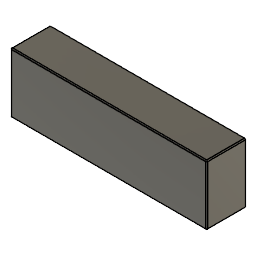
imu_box_v5 (Autodesk Fusion 360 design; units mm, degrees)
Autodesk Fusion 360 part; units mm, degrees
note: some values were not read from the file. Set by a fixed rule: which sketch regions a step uses.
sketch "Sketch1" plane through (0, 0, 0) normal (0, 1, 0) x (1, 0, 0)
  line L0 (0, 0) -> (95, 0)
  line L1 (95, 0) -> (95, -25)
  line L2 (95, -25) -> (0, -25)
  line L3 (0, -25) -> (0, 0)
  line L4 (98, 3) -> (98, -28)
  line L5 (98, -28) -> (-3, -28)
  line L6 (-3, -28) -> (-3, 3)
  line L7 (-3, 3) -> (98, 3)
  dimension "d1" = 95
  dimension "d2" = 25
  dimension "d3" = -3
  constraint horizontal L0
  constraint vertical L1
  constraint horizontal L2
  constraint vertical L3
  constraint coincident L0.start L3.end
  measures "d1" distance of L1.end L2.end
  measures "d2" distance of L0.end L1.end
extrude "Extrude1" add sketch "Sketch1" along normal blind 20 makes body 1
extrude "Extrude2" add sketch "Sketch1" along normal blind 3 contours L0 L1 L2 L3 bodies 1
ref_plane "WorkPlane1" through (47.5, 10, 12.5) normal (0, 0, 1) x (1, 0, 0)
ref_plane "WorkPlane2" through (47.5, 10, 12.5) normal (1, 0, 0) x (0, 0, -1)
sketch "Sketch3" plane through (47.5, 0, 0) normal (1, 0, 0) x (0, 1, 0)
  line L0 (20, 28) -> (0, 28)
  line L1 (0, 28) -> (0, -3)
  line L2 (0, -3) -> (20, -3)
  line L3 (20, -3) -> (20, 0)
  line L4 (20, 0) -> (3, 0)
  line L5 (3, 0) -> (3, 25)
  line L6 (3, 25) -> (20, 25)
  line L7 (20, 25) -> (20, 28)
  circle A0 centre (12.8865, 25) radius 0.75
  circle A1 centre (12.8865, 25) radius 0.9942
  arc A2 (12.1481, 24.8686) -> (20, 21.2966) centre (16.9616, 25.0336) ccw
  arc A3 (13.6365, 25) -> (20, 25) centre (16.8183, 27.2777) ccw
  line L8 (23.2, 12.5) -> (-3.2, 12.5)
  line L9 (20, 28) -> (20, -3)
  line L10 (20, 28) -> (16, 28)
  line L11 (16, 28) -> (16, -3)
  line L12 (20, -3) -> (16, -3)
  arc A4 (20, 0) -> (13.6365, 0) centre (16.8183, -2.2777) ccw
  arc A5 (20, 3.7034) -> (12.1481, 0.1314) centre (16.9616, -0.0336) ccw
  circle A6 centre (12.8865, 0) radius 0.75
  circle A7 centre (12.8865, 0) radius 0.9942
  dimension "d8" = 1.5
  constraint coincident L6 A0.centre
  constraint coincident A0 A2.start
  constraint coincident A0 A3.start
  constraint concentric A0 A1
  constraint coincident L6.end L7.start
  constraint coincident L6 A3.start
  constraint coincident L0.start L7.end
  constraint coincident L2.end L3.start
  constraint coincident A2.end L9
  constraint perpendicular L7 L10
  constraint perpendicular L10 L11
  constraint symmetric A0 L8 A6
  constraint symmetric A1 L8 A7
  constraint symmetric A2.end L8 A5.start
  constraint symmetric A2 L8 A5
  constraint symmetric A3 L8 A4
  constraint symmetric A3.start L8 A4.end
  constraint symmetric A2.start L8 A5.end
  constraint symmetric L8 L6.end L3.end
  measures "d8" diameter of A0
extrude "Extrude9" cut sketch "Sketch3" along normal mid plane 95 contours L6 A1 A3 | L6 A0 A1 | A0 A1 A2 A3 | L6 A0 | L6 A0 | L6 A0 A1 A2 | L4 A5 A6 A7 | L4 A6 A7 | A4 A5 A6 A7 | L4 A4 A7 | L4 A6 | L4 A6 bodies 1
extrude "Extrude10" add sketch "Sketch3" along normal blind 4 from surface at 20 separate body contours A2 A3 L9 L11 | A1 A2 A3 L11 | A0 A1 A2 A3 | L6 A0 | L6 A0 | L9 L11 A4 A5 | L11 A4 A5 A7 | A4 A5 A6 A7 | L4 A6 | L4 A6 makes body 2 at (70.1667, 12.334, 23.6987) makes body 3 at (70.1667, 18.5562, 4.5111)
extrude "Extrude11" add sketch "Sketch3" along normal blind 4 from surface at -20 separate body contours A2 A3 L9 L11 | A1 A2 A3 L11 | A0 A1 A2 A3 | L6 A0 | L6 A0 | L9 L11 A4 A5 | L11 A4 A5 A7 | A4 A5 A6 A7 | L4 A6 | L4 A6 makes body 4 at (30.1667, 18.5562, 4.5111) makes body 5 at (30.1667, 12.334, 23.6987)
extrude "Extrude12" add sketch "Sketch3" along normal mid plane 101 separate body contours L0 L6 L7 L9 L10 L11 | L6 A3 L11 | A2 A3 L9 L11 | A2 L8 L9 L11 | L8 L9 L11 A5 | L9 L11 A4 A5 | L2 L3 L4 L9 L11 L12 | L4 L11 A4 makes body 6
sketch "Sketch8" plane through (0, 16, 0) normal (0, -1, 0) x (1, 0, 0)
  line L0 (-3, -3) -> (98, -3)
  line L1 (98, -3) -> (98, 28)
  line L2 (98, 28) -> (-3, 28)
  line L3 (-3, 28) -> (-3, -3)
  line L4 (0, 10) -> (2.4867, 10)
  line L5 (2.4867, 10) -> (2.4867, 15)
  line L6 (2.4867, 15) -> (0, 15)
  line L7 (0, 15) -> (0, 10)
  line L8 (95, 10) -> (93, 10)
  line L9 (93, 10) -> (93, 15)
  line L10 (93, 15) -> (95, 15)
  line L11 (95, 10) -> (95, 15)
  constraint perpendicular L3 L4
  constraint perpendicular L4 L5
  constraint perpendicular L5 L6
  constraint perpendicular L4 L7
  constraint perpendicular L1 L8
  constraint perpendicular L8 L9
  constraint perpendicular L9 L10
  constraint perpendicular L10 L11
extrude "Extrude13" add sketch "Sketch8" along normal blind 2 contours L4 L5 L6 L7 | L8 L9 L10 L11 bodies 6
fillet "Fillet5" radius 0.5 4 edges at (47.5, 20, 28) (98, 20, 12.5) (47.5, 20, -3) (-3, 20, 12.5) on bodies 6
fillet "Fillet6" radius 1 2 edges at (47.5, 13.8807, 25) (47.5, 13.8807, 0) on bodies 1
fillet "Fillet7" radius 0.5 8 edges at (-3, 10, 28) (-3, 0, 12.5) (-3, 10, -3) (47.5, 0, -3) (47.5, 0, 28) (98, 0, 12.5) (98, 10, -3) (98, 10, 28) on bodies 1
fillet "Fillet8" radius 0.25 2 edges at (47.5, 11.8923, 0) (47.5, 11.8923, 25) on bodies 1
fillet "Fillet9" radius 0.5 4 edges at (47.5, 20, 0) (0, 20, 12.5) (47.5, 20, 25) (95, 20, 12.5) on bodies 1
hidden bodies 2 3 5 4 6
